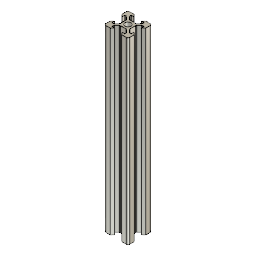
2020_Y_carriage_new_v26 (Autodesk Fusion 360 archive; units mm, degrees)
design "Aluminium profile 149mm"
Autodesk Fusion 360 part; units mm, degrees
sketch "Sketch1" plane through (0, 0, 0) normal (0, 0, 1) x (1, 0, 0)
  circle A0 centre (0, 0) radius 2.5
  arc A1 (-10, -8.5) -> (-8.5, -10) centre (-8.5, -8.5) ccw
  arc A2 (8.5, -10) -> (10, -8.5) centre (8.5, -8.5) ccw
  arc A3 (10, 8.5) -> (8.5, 10) centre (8.5, 8.5) ccw
  arc A4 (-8.5, 10) -> (-10, 8.5) centre (-8.5, 8.5) ccw
  line L0 (-6.987, 5.3) -> (-8, 5.3)
  line L1 (6.987, -5.3) -> (8, -5.3)
  line L2 (8, 5.3) -> (6.987, 5.3)
  line L3 (-8, -5.3) -> (-6.987, -5.3)
  line L4 (-5.3, -8) -> (-5.3, -6.987)
  line L5 (-5.3, 6.987) -> (-5.3, 8)
  line L6 (5.3, 8) -> (5.3, 6.987)
  line L7 (5.3, -6.987) -> (5.3, -8)
  line L8 (2.313, -4) -> (-2.313, -4)
  line L9 (-4, -2.313) -> (-4, 2.313)
  line L10 (-2.313, 4) -> (2.313, 4)
  line L11 (4, 2.313) -> (4, -2.313)
  line L12 (6.2799, -5.0071) -> (4.2929, -3.0201)
  line L13 (5.0071, -6.2799) -> (3.0201, -4.2929)
  line L14 (-5.0071, -6.2799) -> (-3.0201, -4.2929)
  line L15 (-6.2799, -5.0071) -> (-4.2929, -3.0201)
  line L16 (-4.2929, 3.0201) -> (-6.2799, 5.0071)
  line L17 (-3.0201, 4.2929) -> (-5.0071, 6.2799)
  line L18 (3.0201, 4.2929) -> (5.0071, 6.2799)
  line L19 (4.2929, 3.0201) -> (6.2799, 5.0071)
  line L20 (0, -15) -> (0, 19) construction
  line L21 (-20, 0) -> (20, 0) construction
  line L22 (-10, -8.5) -> (-10, -4.75)
  line L23 (-10, 4.75) -> (-10, 8.5)
  line L24 (8.5, -10) -> (4.75, -10)
  line L25 (-4.75, -10) -> (-8.5, -10)
  line L26 (10, 8.5) -> (10, 4.75)
  line L27 (10, -4.75) -> (10, -8.5)
  line L28 (-8.5, 10) -> (-4.75, 10)
  line L29 (4.75, 10) -> (8.5, 10)
  line L30 (5.3, -8) -> (3.1, -8)
  line L31 (-3.1, -8) -> (-5.3, -8)
  line L32 (8, -5.3) -> (8, -3.1)
  line L33 (8, 3.1) -> (8, 5.3)
  line L34 (-5.3, 8) -> (-3.1, 8)
  line L35 (3.1, 8) -> (5.3, 8)
  line L36 (-8, 5.3) -> (-8, 3.1)
  line L37 (-8, -3.1) -> (-8, -5.3)
  line L38 (-4.75, -10) -> (-3.1, -8)
  line L39 (4.75, -10) -> (3.1, -8)
  line L40 (10, -4.75) -> (8, -3.1)
  line L41 (8, 3.1) -> (10, 4.75)
  line L42 (4.75, 10) -> (3.1, 8)
  line L43 (-4.75, 10) -> (-3.1, 8)
  line L44 (-10, 4.75) -> (-8, 3.1)
  line L45 (-10, -4.75) -> (-8, -3.1)
  arc A5 (-5.0071, -6.2799) -> (-5.3, -6.987) centre (-4.3, -6.987) ccw
  arc A6 (5.3, -6.987) -> (5.0071, -6.2799) centre (4.3, -6.987) ccw
  arc A7 (3.0201, -4.2929) -> (2.313, -4) centre (2.313, -5) ccw
  arc A8 (-2.313, -4) -> (-3.0201, -4.2929) centre (-2.313, -5) ccw
  arc A9 (-6.987, -5.3) -> (-6.2799, -5.0071) centre (-6.987, -4.3) ccw
  arc A10 (-4.2929, -3.0201) -> (-4, -2.313) centre (-5, -2.313) ccw
  arc A11 (-4, 2.313) -> (-4.2929, 3.0201) centre (-5, 2.313) ccw
  arc A12 (-6.2799, 5.0071) -> (-6.987, 5.3) centre (-6.987, 4.3) ccw
  arc A13 (6.2799, -5.0071) -> (6.987, -5.3) centre (6.987, -4.3) ccw
  arc A14 (4, -2.313) -> (4.2929, -3.0201) centre (5, -2.313) ccw
  arc A15 (4.2929, 3.0201) -> (4, 2.313) centre (5, 2.313) ccw
  arc A16 (6.987, 5.3) -> (6.2799, 5.0071) centre (6.987, 4.3) ccw
  arc A17 (5.0071, 6.2799) -> (5.3, 6.987) centre (4.3, 6.987) ccw
  arc A18 (2.313, 4) -> (3.0201, 4.2929) centre (2.313, 5) ccw
  arc A19 (-3.0201, 4.2929) -> (-2.313, 4) centre (-2.313, 5) ccw
  arc A20 (-5.3, 6.987) -> (-5.0071, 6.2799) centre (-4.3, 6.987) ccw
  dimension "d3" = 5
  dimension "d4" = 1.5
  dimension "d5" = 16
  dimension "d6" = 10.6
  dimension "d7" = 10.6
  dimension "d8" = 16
  dimension "d23" = 1
  measures "d3" diameter of A0
  measures "d4" radius of A1
  measures "d23" radius of A5
extrude "Extrude1" add sketch "Sketch1" along normal blind 149

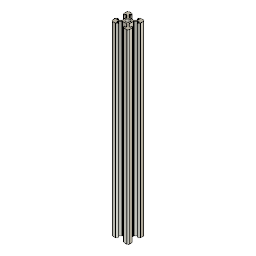
design "Aluminium profile 220mm"
Autodesk Fusion 360 part; units mm, degrees
sketch "Sketch1" plane through (0, 0, 0) normal (0, 0, 1) x (1, 0, 0)
  circle A0 centre (0, 0) radius 2.5
  arc A1 (-10, -8.5) -> (-8.5, -10) centre (-8.5, -8.5) ccw
  arc A2 (8.5, -10) -> (10, -8.5) centre (8.5, -8.5) ccw
  arc A3 (10, 8.5) -> (8.5, 10) centre (8.5, 8.5) ccw
  arc A4 (-8.5, 10) -> (-10, 8.5) centre (-8.5, 8.5) ccw
  line L0 (-6.987, 5.3) -> (-8, 5.3)
  line L1 (6.987, -5.3) -> (8, -5.3)
  line L2 (8, 5.3) -> (6.987, 5.3)
  line L3 (-8, -5.3) -> (-6.987, -5.3)
  line L4 (-5.3, -8) -> (-5.3, -6.987)
  line L5 (-5.3, 6.987) -> (-5.3, 8)
  line L6 (5.3, 8) -> (5.3, 6.987)
  line L7 (5.3, -6.987) -> (5.3, -8)
  line L8 (2.313, -4) -> (-2.313, -4)
  line L9 (-4, -2.313) -> (-4, 2.313)
  line L10 (-2.313, 4) -> (2.313, 4)
  line L11 (4, 2.313) -> (4, -2.313)
  line L12 (6.2799, -5.0071) -> (4.2929, -3.0201)
  line L13 (5.0071, -6.2799) -> (3.0201, -4.2929)
  line L14 (-5.0071, -6.2799) -> (-3.0201, -4.2929)
  line L15 (-6.2799, -5.0071) -> (-4.2929, -3.0201)
  line L16 (-4.2929, 3.0201) -> (-6.2799, 5.0071)
  line L17 (-3.0201, 4.2929) -> (-5.0071, 6.2799)
  line L18 (3.0201, 4.2929) -> (5.0071, 6.2799)
  line L19 (4.2929, 3.0201) -> (6.2799, 5.0071)
  line L20 (0, -15) -> (0, 19) construction
  line L21 (-20, 0) -> (20, 0) construction
  line L22 (-10, -8.5) -> (-10, -4.75)
  line L23 (-10, 4.75) -> (-10, 8.5)
  line L24 (8.5, -10) -> (4.75, -10)
  line L25 (-4.75, -10) -> (-8.5, -10)
  line L26 (10, 8.5) -> (10, 4.75)
  line L27 (10, -4.75) -> (10, -8.5)
  line L28 (-8.5, 10) -> (-4.75, 10)
  line L29 (4.75, 10) -> (8.5, 10)
  line L30 (5.3, -8) -> (3.1, -8)
  line L31 (-3.1, -8) -> (-5.3, -8)
  line L32 (8, -5.3) -> (8, -3.1)
  line L33 (8, 3.1) -> (8, 5.3)
  line L34 (-5.3, 8) -> (-3.1, 8)
  line L35 (3.1, 8) -> (5.3, 8)
  line L36 (-8, 5.3) -> (-8, 3.1)
  line L37 (-8, -3.1) -> (-8, -5.3)
  line L38 (-4.75, -10) -> (-3.1, -8)
  line L39 (4.75, -10) -> (3.1, -8)
  line L40 (10, -4.75) -> (8, -3.1)
  line L41 (8, 3.1) -> (10, 4.75)
  line L42 (4.75, 10) -> (3.1, 8)
  line L43 (-4.75, 10) -> (-3.1, 8)
  line L44 (-10, 4.75) -> (-8, 3.1)
  line L45 (-10, -4.75) -> (-8, -3.1)
  arc A5 (-5.0071, -6.2799) -> (-5.3, -6.987) centre (-4.3, -6.987) ccw
  arc A6 (5.3, -6.987) -> (5.0071, -6.2799) centre (4.3, -6.987) ccw
  arc A7 (3.0201, -4.2929) -> (2.313, -4) centre (2.313, -5) ccw
  arc A8 (-2.313, -4) -> (-3.0201, -4.2929) centre (-2.313, -5) ccw
  arc A9 (-6.987, -5.3) -> (-6.2799, -5.0071) centre (-6.987, -4.3) ccw
  arc A10 (-4.2929, -3.0201) -> (-4, -2.313) centre (-5, -2.313) ccw
  arc A11 (-4, 2.313) -> (-4.2929, 3.0201) centre (-5, 2.313) ccw
  arc A12 (-6.2799, 5.0071) -> (-6.987, 5.3) centre (-6.987, 4.3) ccw
  arc A13 (6.2799, -5.0071) -> (6.987, -5.3) centre (6.987, -4.3) ccw
  arc A14 (4, -2.313) -> (4.2929, -3.0201) centre (5, -2.313) ccw
  arc A15 (4.2929, 3.0201) -> (4, 2.313) centre (5, 2.313) ccw
  arc A16 (6.987, 5.3) -> (6.2799, 5.0071) centre (6.987, 4.3) ccw
  arc A17 (5.0071, 6.2799) -> (5.3, 6.987) centre (4.3, 6.987) ccw
  arc A18 (2.313, 4) -> (3.0201, 4.2929) centre (2.313, 5) ccw
  arc A19 (-3.0201, 4.2929) -> (-2.313, 4) centre (-2.313, 5) ccw
  arc A20 (-5.3, 6.987) -> (-5.0071, 6.2799) centre (-4.3, 6.987) ccw
  dimension "d3" = 5
  dimension "d4" = 1.5
  dimension "d5" = 16
  dimension "d6" = 10.6
  dimension "d7" = 10.6
  dimension "d8" = 16
  dimension "d23" = 1
  measures "d3" diameter of A0
  measures "d4" radius of A1
  measures "d23" radius of A5
extrude "Extrude1" add sketch "Sketch1" along normal blind 220

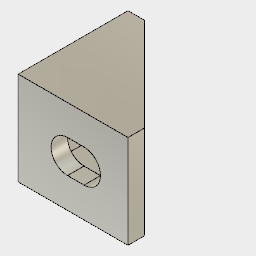
design "corner joint"
Autodesk Fusion 360 part; units mm, degrees
sketch "Sketch1" plane through (0, 0, 0) normal (0, 0, 1) x (1, 0, 0)
  line L0 (0, 0) -> (0, 20)
  line L1 (0, 0) -> (20, 0)
  line L2 (20, 0) -> (20, 3)
  line L3 (0, 20) -> (3, 20)
  line L4 (3, 20) -> (20, 3)
  line L5 (3, 20) -> (3, 0)
  line L6 (20, 3) -> (0, 3)
  dimension "d1" = 20
  dimension "d2" = 20
  dimension "d3" = 3
  dimension "d4" = 3
  constraint coincident L0.start L1.start
  constraint coincident L1 L0.start
  constraint perpendicular L1 L5
  constraint coincident L0 L1.start
  constraint perpendicular L0 L6
extrude "Extrude1" add sketch "Sketch1" along normal blind 3
extrude "Extrude2" add sketch "Sketch1" along normal blind 17 contours L0 L1 L5 L6 | L0 L3 L5 L6 | L1 L2 L5 L6
extrude "Extrude3" add sketch "Sketch1" against normal blind 3 from surface at 17
sketch "Sketch2" plane through (0, 0, 0) normal (0, -1, 0) x (1, 0, 0)
  line L0 (0, 17) -> (0, 0)
  line L1 (0, 0) -> (20, 0)
  line L2 (20, 0) -> (20, 17)
  line L3 (20, 17) -> (0, 17)
  line L4 (9, 5.5) -> (12, 5.5)
  arc A0 (12, 5.5) -> (12, 11.5) centre (12, 8.5) ccw
  line L5 (12, 11.5) -> (9, 11.5)
  arc A1 (9, 11.5) -> (9, 5.5) centre (9, 8.5) ccw
  line L6 (9, 8.5) -> (12, 8.5) construction
  dimension "d12" = 6
  dimension "d15" = 8.5
  dimension "d16" = 9
  dimension "d17" = 3
  constraint tangent L4 A0
  constraint tangent A0 L5
  constraint parallel L4 L5
  constraint tangent L5 A1
  constraint tangent L4 A1
  constraint perpendicular L0 L6
  measures "d12" diameter of A0
sketch "Sketch3" plane through (0, 0, 0) normal (-1, 0, 0) x (0, -1, 0)
  line L0 (-20, 17) -> (-20, 0)
  line L1 (-20, 0) -> (0, 0)
  line L2 (0, 0) -> (0, 17)
  line L3 (0, 17) -> (-20, 17)
  line L4 (-12, 5.5) -> (-9, 5.5)
  arc A0 (-9, 5.5) -> (-9, 11.5) centre (-9, 8.5) ccw
  line L5 (-9, 11.5) -> (-12, 11.5)
  arc A1 (-12, 11.5) -> (-12, 5.5) centre (-12, 8.5) ccw
  line L6 (-12, 8.5) -> (-9, 8.5) construction
  dimension "d13" = 3
  dimension "d14" = 6
  dimension "d18" = 8.5
  dimension "d19" = 9
  constraint tangent L4 A0
  constraint tangent A0 L5
  constraint parallel L4 L5
  constraint tangent L5 A1
  constraint tangent L4 A1
  constraint perpendicular L0 L6
  measures "d14" diameter of A0
extrude "Extrude4" cut sketch "Sketch3" against normal through all contours L4 A0 L5 A1
extrude "Extrude5" cut sketch "Sketch2" against normal through all contours L4 A0 L5 A1
